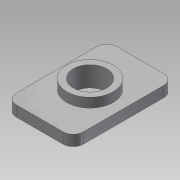
# Autodesk Inventor part: 5mm Tee Nut
Saved by Autodesk Inventor 2013 SP2 (Build 170200200, 200)
## iProperties
Created: 2013-06-22
Part Number: 5mm Tee Nut
Material: Steel
Document SubType Name: Modeling
Designer: Jon Hollander
Density: 7.85 g/cm^3
Mass: 1.80829 g
Surface Area: 4.10219 cm^2
Volume: 0.230355 cm^3
Author: Jon Hollander
Autodesk Inventor part; units mm, degrees
ref_plane "YZ Plane" through (0, 0, 0) normal (1, 0, 0) x (0, 1, 0)
ref_plane "XZ Plane" through (0, 0, 0) normal (0, 1, 0) x (-1, 0, 0)
ref_plane "XY Plane" through (0, 0, 0) normal (0, 0, 1) x (1, 0, 0)
sketch "Sketch1" plane through (0, 0, 0) normal (0, 0, 1) x (1, 0, 0)
  line L0 (-5, 7.5) -> (5, 7.5)
  line L1 (5, 7.5) -> (5, -7.5)
  line L2 (5, -7.5) -> (-5, -7.5)
  line L3 (-5, -7.5) -> (-5, 7.5)
  line L4 (-5, 7.5) -> (5, -7.5) construction
  line L5 (5, 7.5) -> (-5, -7.5) construction
  point P0 (0, 0)
  dimension "d0" = 10
  dimension "d1" = 15
  constraints: 12 end point, 2 midpoint, 2 parallel, 1 horizontal, 1 perpendicular
  measures "d0" distance of L1.end L2.end
  measures "d1" distance of L0.end L1.end
extrude "Extrusion1" add sketch "Sketch1" along normal blind 1.6
sketch "Sketch2" plane through (0, 0, 1.6) normal (0, 0, 1) x (1, 0, 0)
  circle A0 centre (0, 0) radius 3.45
  dimension "d4" = 6.9
  constraints: 1 centre point, 1 coincident
  measures "d4" diameter of A0
extrude "Extrusion2" add sketch "Sketch2" along normal blind 1.4
sketch "Sketch3" plane through (0, 0, 3) normal (0, 0, 1) x (1, 0, 0)
  circle A0 centre (0, 0) radius 3.45 projected
  constraints: 1 coincident
hole "Hole1" at (0, 0, 3) direction (0, 0, -1) diameter 5 end through all
fillet "Fillet1" radius 1.5 4 edges at (5, 7.5, 0.8) (-5, 7.5, 0.8) (5, -7.5, 0.8) (-5, -7.5, 0.8)
body "Solid1"
